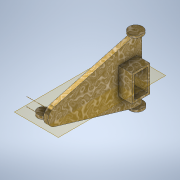
# Autodesk Inventor part: design base robot
Saved by Autodesk Inventor 2022 (Build 260153000, 153)
## iProperties
Created: 2021-07-07
Part Number: design base robot
Material: Generic
Document SubType Name: Sheet Metal
Designer: Nay
Density: 1 g/cm^3
Sheet Metal Rule: Default_mm
Appearance: Default
Author: Nay
Autodesk Inventor part; units mm, degrees
ref_plane "YZ Plane" through (0, 0, 0) normal (1, 0, 0) x (0, 1, 0)
ref_plane "XY Plane" through (0, 0, 0) normal (0, 0, 1) x (1, 0, 0)
sketch "Sketch1" plane through (0, 0, 0) normal (1, 0, 0) x (0, 1, 0)
  line L0 (7.5, -11.76) -> (-7.5, -11.76)
  line L1 (-7.5, -11.76) -> (0.39, 14.64)
  line L2 (0.39, 14.64) -> (7.5, -11.76)
  point P0 (0, 0)
  dimension "d0" = 15
  dimension "d1" = 7.5
  constraints: 6 end point, 1 horizontal
  measures "d0" distance of L0.start L0.end
  measures "d1" horizontal distance of point (0, 0) L0.start
extrude "Extrusion1" add sketch "Sketch1" along normal blind 1
fillet "Fillet1" radius 2 1 edges at (0.5, 0.39, 14.64)
sketch "Sketch2" plane through (1, 0, 0) normal (1, 0, 0) x (0, 0, -1)
  line L0 (11.76, -7.5) -> (11.76, 7.5) projected
  line L1 (11.76, 7) -> (1.6086, 7)
  line L2 (11.76, -7) -> (0.4021, -7)
  line L3 (11.76, 7.5) -> (-7.8408, 2.2211) projected
  line L4 (9.9035, 7) -> (11.76, 7.5)
  line L5 (11.76, 7.5) -> (11.76, 7)
  line L6 (11.76, -7) -> (11.76, -7.5)
  line L7 (11.76, -7.5) -> (10.087, -7)
  line L8 (-7.8934, -1.6263) -> (11.76, -7.5) projected
  line L9 (11.76, -7) -> (11.76, -7.5)
  point P0 (0, 0)
  dimension "d5" = 0.5
  dimension "d6" = 0.5
  constraints: 14 end point, 6 point on line, 3 collinear, 2 horizontal
  measures "d5" distance of L1.start L0.end
  measures "d6" distance from line of L0.start L2
extrude "Extrusion2" cut sketch "Sketch2" against normal blind 1 contours L1 L3 L0
sketch "Sketch3" plane through (1, 0, 0) normal (1, 0, 0) x (0, 0, -1)
  line L0 (11.76, -7.5) -> (11.76, 7) projected
  line L1 (11.76, -7) -> (8.3926, -7)
  line L2 (-7.8934, -1.6263) -> (11.76, -7.5) projected
  line L3 (10.087, -7) -> (11.76, -7.5)
  line L4 (11.76, -7.5) -> (11.76, -7)
  point P0 (0, 0)
  dimension "d9" = 0.5
  constraints: 6 end point, 3 point on line, 1 collinear, 1 horizontal
  measures "d9" distance from line of L0.start L1
extrude "Extrusion3" cut sketch "Sketch3" against normal blind 1
sketch "Sketch6" plane through (1, 0, 0) normal (1, 0, 0) x (0, 0, -1)
  line L0 (10.587, -7) -> (10.587, 7) projected
  line L1 (10.587, -3) -> (6.587, -3)
  line L2 (6.587, -3) -> (6.587, 3)
  line L3 (6.587, 3) -> (10.587, 3)
  line L4 (10.587, 3) -> (10.587, -3)
  point P0 (0, 0)
  dimension "d20" = 6
  dimension "d21" = 4
  dimension "d22" = 3
  constraints: 8 end point, 2 parallel, 1 horizontal, 1 perpendicular, 1 point on line
  measures "d20" distance of L1.end L2.end
  measures "d21" distance of L1.start L1.end
  measures "d22" distance from line of point (0, 0) L1
extrude "Extrusion6" add sketch "Sketch6" along normal blind 3
sketch "Sketch7" plane through (4, 0, 0) normal (1, 0, 0) x (0, 0, -1)
  line L0 (10.087, -2.5) -> (7.087, -2.5)
  line L1 (7.087, -2.5) -> (7.087, 2.5)
  line L2 (7.087, 2.5) -> (10.087, 2.5)
  line L3 (10.087, 2.5) -> (10.087, -2.5)
  line L4 (10.587, -3) -> (10.587, 3) projected
  point P0 (0, 0)
  dimension "d25" = 3
  dimension "d26" = 5
  dimension "d27" = 2.5
  dimension "d28" = 0.5
  constraints: 8 end point, 2 parallel, 1 horizontal, 1 perpendicular
  measures "d25" distance of L0.start L0.end
  measures "d26" distance of L0.end L1.end
  measures "d27" distance from line of point (0, 0) L0
  measures "d28" distance between parallel lines of L4 L3
extrude "Extrusion7" cut sketch "Sketch7" against normal blind 3
sketch "Sketch8" plane through (0, -1.6263, 7.8934) normal (0, -0.9581254, 0.2863488) x (1, 0, 0)
  point P0 (0, -7.0972)
sketch "Sketch9" plane through (1, 7, -9.9035) normal (0, 1, 0) x (1, 0, 0)
  circle A0 centre (-0.5, 1) radius 1.5
  line L0 (0, 0) -> (-1, 0) projected
  line L1 (-1, 0) -> (-1, 1.8565) projected
  point P0 (-1, -9.9035)
  dimension "d32" = 3
  dimension "d33" = 1
  dimension "d34" = 0.5
  constraints: 1 centre point
  measures "d32" diameter of A0
  measures "d33" distance from line of A0.centre L0
  measures "d34" distance from line of L1 A0.centre
extrude "Extrusion8" add sketch "Sketch9" along normal blind 0.5
sketch "Sketch10" plane through (1, -7, -11.76) normal (0, -1, 0) x (1, 0, 0)
  circle A0 centre (-0.5, 0.673) radius 1.5
  line L0 (-1, 1.673) -> (0, 1.673) projected
  line L1 (0, 1.673) -> (0, 0) projected
  point P0 (-1, 11.76)
  dimension "d37" = 3
  dimension "d38" = 1
  dimension "d39" = 0.5
  constraints: 1 centre point
  measures "d37" diameter of A0
  measures "d38" distance from line of L0 A0.centre
  measures "d39" distance from line of L1 A0.centre
extrude "Extrusion9" add sketch "Sketch10" along normal blind 0.5
sketch "Sketch11" plane through (0, 0, 0) normal (-1, 0, 0) x (0, 0, 1)
  circle A0 centre (8.037, 1.3078) radius 0.05
  circle A1 centre (8.0284, -0.6921) radius 0.05
  point P0 (0, 0)
  dimension "d42" = 0.1
  dimension "d43" = 0.1
  dimension "d44" = 2
  constraints: 2 centre point
  measures "d42" diameter of A0
  measures "d43" diameter of A1
  measures "d44" distance of A0.centre A1.centre
extrude "Extrusion10" add sketch "Sketch11" along normal blind 5
sketch "Sketch12" plane through (0, 0, 0) normal (-1, 0, 0) x (0, 0, 1)
  point P0 (0, 0)
ref_plane "Work Plane1" through (0, -0.7421, 8.0284) normal (0, 1, 0) x (-1, 0, 0)
sketch "Sketch13" plane through (0, 0, 0) normal (0, 1, 0) x (-1, 0, 0)
  line L0 (0, 8.087) -> (5, 8.087) projected
  circle A0 centre (1.2639, 8.087) radius 1.2639
  line L1 (0, 9.3207) -> (0, 7.8408) projected
  point P0 (0, 0)
  point P1 (0, 7.8934)
  constraints: 1 centre point, 1 point on line, 1 tangent
extrude "Extrusion11" add sketch "Sketch13" along normal mid plane 0.75
equation "\"GapSize\" = Thickness"
equation "\"BendRadius\" = Thickness"
equation "\"MinimumRemnant\" = 2 * Thickness"
equation "\"BendReliefDepth\" = 0.5 * Thickness"
equation "\"BendReliefWidth\" = Thickness"
equation "\"CornerReliefSize\" = 4 * Thickness"
equation "\"JacobiRadiusSize\" = BendRadius"
equation "\"TransitionRadius\" = BendRadius"
equation "\"Thickness\" = 0.5"
body "Solid1"
